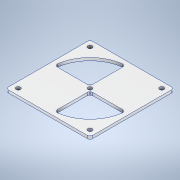
# Autodesk Inventor part: Feeder Bottom Plate
Saved by Autodesk Inventor 2020.3 (Build 243373000, 373)
## iProperties
Created: 2020-07-23
Part Number: Feeder Bottom Plate
Material: Aluminum 6061
Document SubType Name: Modeling
Designer: juanp
Density: 2.7 g/cm^3
Appearance: Aluminum - Flat
Author: juanp
Autodesk Inventor part; units mm, degrees
ref_plane "YZ Plane" through (0, 0, 0) normal (1, 0, 0) x (0, 1, 0)
ref_plane "XZ Plane" through (0, 0, 0) normal (0, 1, 0) x (-1, 0, 0)
ref_plane "XY Plane" through (0, 0, 0) normal (0, 0, 1) x (1, 0, 0)
sketch "Sketch1" plane through (0, 0, 0) normal (0, 1, 0) x (-1, 0, 0)
  circle A0 centre (0, 0) radius 30 construction
  line L0 (-30, 0) -> (0, 0) construction
  line L1 (0, 30) -> (0, 0) construction
  line L2 (0, 0) -> (0, -30) construction
  line L3 (0, 0) -> (30, 0) construction
  arc A1 (27, 0) -> (-1.5, 26.9583) centre (0, 0) ccw construction
  circle A2 centre (0, 0) radius 1.5
  circle A3 centre (0, 0) radius 3
  line L4 (-1.5, 2.5981) -> (-1.5, 26.9583)
  line L5 (1.5, 26.9583) -> (1.5, 2.5981) construction
  line L6 (-1.5, 14.7782) -> (1.5, 14.7782) construction
  line L7 (-2.5981, -1.5) -> (-26.9583, -1.5) construction
  line L8 (-26.9583, 1.5) -> (-2.5981, 1.5)
  line L9 (1.5, -2.5981) -> (1.5, -26.9583)
  line L10 (-1.5, -26.9583) -> (-1.5, -2.5981) construction
  line L11 (2.5981, 1.5) -> (26.9583, 1.5) construction
  line L12 (26.9583, -1.5) -> (2.5981, -1.5)
  line L13 (1.5, -26.9583) -> (1.5, -29.9625) construction
  line L14 (26.9583, -1.5) -> (29.9625, -1.5) construction
  line L15 (30, 30) -> (-30, 30)
  line L16 (-30, 30) -> (-30, -30)
  line L17 (-30, -30) -> (30, -30)
  line L18 (30, -30) -> (30, 30)
  line L19 (30, 30) -> (21.2132, 21.2132) construction
  line L20 (-30, 30) -> (-21.2132, 21.2132) construction
  line L21 (21.2132, 21.2132) -> (-21.2132, -21.2132) construction
  line L22 (21.2132, -21.2132) -> (30, -30) construction
  line L23 (-21.2132, -21.2132) -> (-30, -30) construction
  line L24 (-21.2132, 21.2132) -> (21.2132, -21.2132) construction
  circle A4 centre (-25.6066, 25.6066) radius 1.55
  circle A5 centre (-25.6066, -25.6066) radius 1.55
  circle A6 centre (25.6066, -25.6066) radius 1.55
  circle A7 centre (25.6066, 25.6066) radius 1.55
  arc A8 (26.9583, -1.5) -> (27, 0) centre (0, 0) ccw construction
  arc A9 (0, -27) -> (26.9583, -1.5) centre (0, 0) ccw
  arc A10 (-1.5, 26.9583) -> (-26.9583, 1.5) centre (0, 0) ccw
  arc A11 (-26.9583, 1.5) -> (0, -27) centre (0, 0) ccw construction
  point P0 (0, 14.7782)
  point P1 (-14.7782, -1.5)
  point P2 (-14.7782, 1.5)
  point P3 (1.5, -14.7782)
  point P4 (-1.5, -14.7782)
  point P5 (14.7782, 1.5)
  point P6 (14.7782, -1.5)
  dimension "d5" = 60
  dimension "d6" = 3
  dimension "d7" = 3
  dimension "d8" = 6
  dimension "d9" = 360
  dimension "d10" = 3
  dimension "d14" = 3.1
  dimension "d15" = 3.1
  dimension "d16" = 3.1
  dimension "d17" = 3.1
  constraints: 50 end point, 15 point on circle, 11 centre point, 9 midpoint, 6 horizontal, 6 perpendicular, 5 coincident, 5 point on line, 5 vertical, 2 parallel, 45 other
  measures "d7" diameter of A2
  measures "d8" diameter of A3
  measures "d10" distance between parallel lines of L5 L4
  measures "d14" diameter of A4
  measures "d15" diameter of A5
  measures "d16" diameter of A6
  measures "d17" diameter of A7
extrude "Extrusion1" add sketch "Sketch1" along normal blind 2 contours A3 | L18 L17 L16 L15
fillet "Fillet1" radius 2 4 edges at (-30, 1, 30) (30, 1, 30) (30, 1, -30) (-30, 1, -30)
fillet "Fillet2" radius 2 8 edges at (1.5, 1, 26.9583) (26.9583, 1, 1.5) (1.5, 1, 2.5981) (2.5981, 1, 1.5) (-2.5981, 1, -1.5) (-1.5, 1, -2.5981) (-26.9583, 1, -1.5) (-1.5, 1, -26.9583)
body "Solid1"
